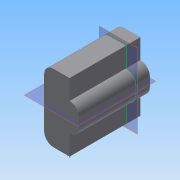
# Autodesk Inventor part: head2
Saved by Autodesk Inventor 2015 (Build 190159000, 159)
## iProperties
Created: 2015-06-18
Part Number: head2
Material: Générique
Document SubType Name: Modeling
Designer: Gregwar
Density: 1 g/cm^3
Appearance: Par défaut
Author: Gregwar
Autodesk Inventor part; units mm, degrees
ref_plane "YZ Plane" through (0, 0, 0) normal (1, 0, 0) x (0, 1, 0)
ref_plane "XZ Plane" through (0, 0, 0) normal (0, 1, 0) x (-1, 0, 0)
ref_plane "XY Plane" through (0, 0, 0) normal (0, 0, 1) x (1, 0, 0)
sketch "Esquisse1" plane through (0, 0, 0) normal (0, 1, 0) x (-1, 0, 0)
  line L0 (0, 0) -> (27, 0)
  line L1 (27, 0) -> (27, -72)
  line L2 (27, -72) -> (0, -72)
  line L3 (0, -72) -> (0, 0)
  line L4 (0, -21) -> (-10, -21)
  line L5 (-10, -21) -> (-10, -51)
  line L6 (-10, -51) -> (0, -51)
  line L7 (0, -51) -> (0, -21)
  point P0 (0, -36)
  dimension "d0" = 27
  dimension "d1" = 72
  dimension "d2" = 30
  dimension "d3" = 10
  constraints: 16 end point, 4 parallel, 2 horizontal, 2 midpoint, 2 perpendicular
  measures "d0" distance of L0.start L0.end
  measures "d1" distance of L0.end L1.end
  measures "d2" distance of L4.end L5.end
  measures "d3" distance of L5.end L6.end
extrude "Extrusion1" add sketch "Esquisse1" along normal blind 75
sketch "Esquisse2" plane through (0, 75, 0) normal (0, 1, 0) x (1, 0, 0)
  line L0 (0, 21) -> (10, 21) construction
  line L1 (10, 21) -> (10, 51) construction
  line L2 (10, 51) -> (0, 51) construction
  line L3 (0, 51) -> (0, 72) construction
  line L4 (0, 72) -> (-27, 72) construction
  line L5 (-27, 72) -> (-27, 0) construction
  line L6 (-27, 0) -> (0, 0) construction
  line L7 (0, 0) -> (0, 21) construction
  line L8 (-27, 72) -> (-27, 0) construction
  line L9 (-27, 72) -> (-27, 0) construction
  line L10 (-27, 36) -> (10, 36) construction
  circle A0 centre (-14.5005, 20.2664) radius 7.6563
  circle A1 centre (-14.5005, 51.7336) radius 7.6563
  line L11 (1.4504, 25.5678) -> (1.4504, 47.6136)
  line L12 (1.4504, 25.5678) -> (7.5686, 36) construction
  line L13 (7.5686, 36) -> (1.4504, 47.6136) construction
  spline S0 degree 2 poles (1.4504, 25.5678) (7.5686, 36) (1.4504, 47.6136) knots 1 1 1 2 2 2
  dimension "d28" = 15.3126
  constraints: 4 end point, 2 centre point, 2 midpoint, 1 point on line, 1 symmetric about line, 1 vertical, 4 other
  measures "d28" diameter of A0
extrude "Extrusion2" cut sketch "Esquisse2" against normal blind 2
fillet "Congé1" radius 10 2 edges at (-27, 37.5, -72) (-27, 37.5, 0)
fillet "Congé2" radius 10 2 edges at (10, 37.5, -51) (10, 37.5, -21)
ref_plane "Plan de construction1" through (0, 60, 0) normal (0, 1, 0) x (1, 0, 0)
sketch "Esquisse3" plane through (0, 0, -72) normal (0, 0, -1) x (-1, 0, 0)
  point P0 (0, 0)
sketch "Esquisse4" plane through (0, 60, 0) normal (0, 1, 0) x (1, 0, 0)
  arc A0 (0, 21) -> (10, 31) centre (0, 31) ccw projected
  line L0 (10, 31) -> (10, 41) projected
  arc A1 (10, 41) -> (0, 51) centre (0, 41) ccw projected
  line L1 (0, 51) -> (0, 72) projected
  line L2 (0, 72) -> (-17, 72) projected
  arc A2 (-17, 72) -> (-27, 62) centre (-17, 62) ccw projected
  line L3 (-27, 62) -> (-27, 10) projected
  arc A3 (-27, 10) -> (-17, 0) centre (-17, 10) ccw projected
  line L4 (-17, 0) -> (0, 0) projected
  line L5 (0, 0) -> (0, 21) projected
  circle A4 centre (-14.5005, 20.2664) radius 7.6563 projected
  line L6 (1.4504, 25.5678) -> (1.4504, 47.6136) projected
  circle A5 centre (-14.5005, 51.7336) radius 7.6563 projected
  line L7 (0, 72) -> (-17, 72) projected
  line L8 (-14.5005, 72) -> (-37.6894, 78.8251)
  line L9 (-37.6894, 78.8251) -> (-26.0949, 60.5542)
  line L10 (-26.0949, 60.5542) -> (-14.5005, 72)
  constraints: 6 end point, 3 point on line, 1 vertical alignment
ref_plane "Plan de construction2" through (0, 0, -36) normal (0, 0, -1) x (-1, 0, 0)
